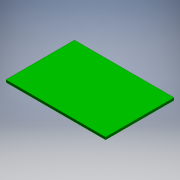
# Autodesk Inventor part: TFT_kiban
Saved by Autodesk Inventor 2016 (Build 200138000, 138)
## iProperties
Created: 2016-09-20
Part Number: TFT_kiban
Material: 一般
Document SubType Name: Modeling
Designer: KOTA-NPC2
Density: 1 g/cm^3
Appearance: 既定
Author: KOTA-NPC2
Autodesk Inventor part; units mm, degrees
ref_plane "YZ Plane" through (0, 0, 0) normal (1, 0, 0) x (0, 1, 0)
ref_plane "XZ Plane" through (0, 0, 0) normal (0, 1, 0) x (-1, 0, 0)
ref_plane "XY Plane" through (0, 0, 0) normal (0, 0, 1) x (1, 0, 0)
sketch "スケッチ1" plane through (0, 0, 0) normal (0, 0, 1) x (1, 0, 0)
  line L0 (-24.75, 17) -> (24.75, 17)
  line L1 (24.75, 17) -> (24.75, -17)
  line L2 (24.75, -17) -> (-24.75, -17)
  line L3 (-24.75, -17) -> (-24.75, 17)
  point P0 (0, 0)
  dimension "d2" = 17
  dimension "d3" = 24.75
  dimension "d4" = 17
  dimension "d5" = 24.75
  constraints: 8 end point, 2 parallel, 1 horizontal, 1 perpendicular
  measures "d2" distance from line of point (0, 0) L0
  measures "d3" distance from line of point (0, 0) L1
  measures "d4" distance from line of L2 point (0, 0)
  measures "d5" distance from line of point (0, 0) L3
extrude "押し出し5" add sketch "スケッチ1" against normal blind 1.2
equation "\"d4\" = d2"
equation "\"d5\" = d3"
